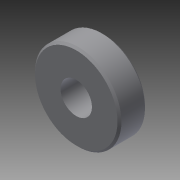
# Autodesk Inventor part: 608
Saved by Autodesk Inventor 2013 (Build 170138000, 138)
## iProperties
Created: 2014-03-03
Part Number: 608
Material: Generic
Document SubType Name: Modeling
Designer: employee
Density: 1 g/cm^3
Author: employee
Autodesk Inventor part; units mm, degrees
ref_plane "YZ Plane" through (0, 0, 0) normal (1, 0, 0) x (0, 1, 0)
ref_plane "XZ Plane" through (0, 0, 0) normal (0, 1, 0) x (-1, 0, 0)
ref_plane "XY Plane" through (0, 0, 0) normal (0, 0, 1) x (1, 0, 0)
sketch "Sketch1" plane through (0, 0, 0) normal (0, 0, 1) x (1, 0, 0)
  line L0 (0, 0) -> (4, 0)
  line L1 (4, 0) -> (4, 7)
  line L2 (4, 7) -> (10.5, 7)
  line L3 (11, 6.5) -> (11, 0.5)
  line L4 (10.5, 0) -> (4, 0)
  line L5 (11, 6.5) -> (10.5, 7)
  line L6 (11, 0.5) -> (10.5, 0)
  line L7 (0, -1.4) -> (0, 8.4) projected
  point P0 (11, 7)
  point P1 (11, 0)
  dimension "d0" = 0.5
  dimension "d1" = 0.5
  dimension "d2" = 0.5
  dimension "d3" = 0.5
  dimension "d4" = 4
  dimension "d5" = 11
  dimension "d6" = 7
  constraints: 14 end point, 4 point on line, 2 parallel, 1 collinear, 1 horizontal, 1 perpendicular
  measures "d0" distance of L3.start point (11, 7)
  measures "d1" distance of L2.end point (11, 7)
  measures "d2" distance of L3.end point (11, 0)
  measures "d3" distance of L4.start point (11, 0)
  measures "d4" distance of L0.start L0.end
  measures "d5" distance from line of L3 L0.start
  measures "d6" distance of L0.end L1.end
revolve "Revolution1" add sketch "Sketch1" angle 360 about axis through (0, -10, 0) along (0, 1, 0)
equation "\"d1\" = d0"
equation "\"d2\" = d0"
equation "\"d3\" = d2"
body "Solid1"
